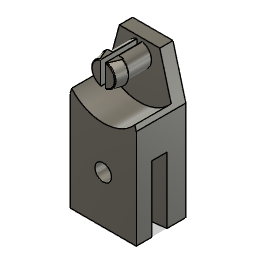
22mm Bearing Clips v7 (Autodesk Fusion 360 design; units mm, degrees)
Autodesk Fusion 360 part; units mm, degrees
sketch "Sketch1" plane through (0, 0, 0) normal (0, 0, 1) x (1, 0, 0)
  line L0 (-10, 15) -> (10, 15) construction
  line L1 (10, 15) -> (10, -15)
  line L2 (10, -15) -> (-10, -15)
  line L3 (-10, -15) -> (-10, 15)
  line L4 (-10, 15) -> (10, -15) construction
  line L5 (-10, 15) -> (-6.1006, 29.4352)
  line L6 (-6.1006, 29.4352) -> (6.1006, 29.4352)
  line L7 (6.1006, 29.4352) -> (10, 15)
  dimension "d1" = 30
  dimension "d2" = 20
  constraint horizontal L0
  constraint vertical L1
  constraint horizontal L2
  constraint vertical L3
  constraint midpoint origin L4
  constraint perpendicular L3 L6
  constraint equal L5 L7
  measures "d1" distance of L0.start L2.end
  measures "d2" distance of L0.start L0.end
extrude "Extrude1" add sketch "Sketch1" along normal blind 15
sketch "Sketch3" plane through (0, 0, 15) normal (0, 0, 1) x (1, 0, 0)
  line L0 (6.1006, 29.4352) -> (-6.1006, 29.4352)
  line L1 (-6.1006, 29.4352) -> (-10, 15)
  line L2 (-10, 15) -> (-10, -15)
  line L3 (-10, -15) -> (10, -15)
  line L4 (10, -15) -> (10, 15)
  line L5 (10, 15) -> (6.1006, 29.4352)
  circle A0 centre (0, 25) radius 11
  circle A1 centre (0, 25) radius 12.75
  line L6 (-0.75, 15.25) -> (0.75, 15.25)
  line L7 (0.75, 15.25) -> (0.75, 34.75)
  line L8 (0.75, 34.75) -> (-0.75, 34.75)
  line L9 (-0.75, 34.75) -> (-0.75, 15.25)
  line L10 (0.75, 34.75) -> (-0.75, 15.25)
  dimension "d7" = 22
  dimension "d8" = 1.75
  dimension "d18" = 1.5
  constraint horizontal L6
  constraint vertical L7
  constraint horizontal L8
  constraint vertical L9
  constraint midpoint A0.centre L10
  measures "d7" diameter of A0
  measures "d18" distance of L6.start L6.end
extrude "Extrude3" cut sketch "Sketch3" against normal blind 11 contours L0 L1 L5 A0 L6 L7 L9 | L0 L6 L7 L10 | L1 L5 A0 A1 | L0 L9 L10 picked at (-0.8699, 12.8858)
sketch "Sketch4" plane through (0, 0, 15) normal (0, 0, 1) x (1, 0, 0)
  circle A0 centre (0, 25) radius 3.6
  line L0 (0, 28.6) -> (0, 21.4)
  dimension "d12" = 7.2
  constraint coincident A0 L0.start
  constraint coincident A0 L0.end
  constraint vertical L0
  measures "d12" diameter of A0
extrude "Extrude4" add sketch "Sketch4" against normal blind 11 contours A0 L0 picked at (-2.3666, 24.8227)
sketch "Sketch5" plane through (0, 0, 0) normal (1, 0, 0) x (0, 0, -1)
  line L0 (-15, 28.6) -> (-15, 21.4)
  line L1 (-15, 21.4) -> (-4, 21.4)
  line L2 (-4, 21.4) -> (-4, 28.6)
  line L3 (-4, 28.6) -> (-15, 28.6)
  line L4 (-15, 28.6) -> (-11.226, 29.35)
  line L5 (-11.226, 29.35) -> (-11.226, 28.6)
  dimension "d21" = 0.75
  constraint coincident L3 L5.end
  constraint perpendicular L3 L5
  constraint coincident L0.start L3.end
  measures "d21" distance of L4.end L5.end
revolve "Revolve1" add sketch "Sketch5" angle 360 about axis through (0, 25, 15) along (0, 0, 1) contours L3 L4 L5
extrude "Extrude5" add sketch "Sketch4" against normal blind 11 contours A0 L0 picked at (0.4985, 23.9084)
extrude "Extrude6" cut sketch "Sketch3" against normal blind 11 contours L0 L6 L7 L10 | L0 L9 L10
fillet "Fillet1" radius 0.35 1 edges at (4.35, 25, 11.226)
fillet "Fillet1" radius 0.35 1 edges at (-4.35, 25, 11.226)
fillet "Fillet2" radius 0.25 1 edges at (-3.6, 25, 15)
fillet "Fillet2" radius 0.25 1 edges at (3.6, 25, 15)
sketch "Sketch6" plane through (10, 0, 0) normal (1, 0, 0) x (0, 0, -1)
  line L0 (-15, -15) -> (0, -15)
  line L1 (0, -15) -> (0, 15)
  line L2 (0, 15) -> (-15, 15)
  line L3 (-15, 15) -> (-15, -15)
  line L4 (-4, 28.5) -> (-15, 28.5)
  line L5 (-15, 28.5) -> (-15, 29.5)
  line L6 (-15, 29.5) -> (-4, 29.5)
  line L7 (-4, 29.5) -> (-4, 28.5)
  line L8 (-4, 21.5) -> (-15, 21.5)
  line L9 (-15, 21.5) -> (-15, 20.5)
  line L10 (-15, 20.5) -> (-4, 20.5)
  line L11 (-4, 20.5) -> (-4, 21.5)
  constraint horizontal L4
  constraint vertical L5
  constraint horizontal L6
  constraint vertical L7
  constraint horizontal L8
  constraint vertical L9
  constraint horizontal L10
  constraint vertical L11
extrude "Extrude7" cut sketch "Sketch6" against normal blind 15 contours L4 L5 L6 L7 | L8 L9 L10 L11
sketch "Sketch7" plane through (0, 0, 0) normal (0, 1, 0) x (1, 0, 0)
  line L0 (-10.0845, -5.713) -> (-10.0845, -10.2645)
  line L1 (10, -10.2768) -> (10, -5.7262)
  arc A0 (-10.0845, -5.713) -> (10, -5.7262) centre (0, 58.5) ccw
  arc A1 (-10.0845, -10.2645) -> (10, -10.2768) centre (0, 58.5) ccw
  dimension "d32" = 130
  dimension "d38" = 69.5
  constraint vertical L0
  constraint vertical L1
  measures "d32" diameter of A0
  measures "d38" radius of A1
extrude "Extrude8" cut sketch "Sketch7" against normal blind 15
extrude "Extrude9" cut sketch "Sketch7" along normal blind 5
hole "Hole1" at (0, -0.6705, 15) direction (0, 0, -1) diameter 5 depth 15 tip angle 118
